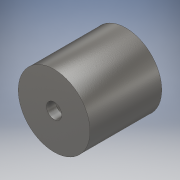
# Autodesk Inventor part: SensorHalter
Saved by Autodesk Inventor 2018.3 (Build 223284000, 284)
## iProperties
Created: 2020-01-09
Part Number: SensorHalter
Material: Generisch
Document SubType Name: Modeling
Designer: DerLobre
Density: 1 g/cm^3
Appearance: Galvanisiert
Author: DerLobre
Autodesk Inventor part; units mm, degrees
ref_plane "YZ Plane" through (0, 0, 0) normal (1, 0, 0) x (0, 1, 0)
ref_plane "XZ Plane" through (0, 0, 0) normal (0, 1, 0) x (-1, 0, 0)
ref_plane "XY Plane" through (0, 0, 0) normal (0, 0, 1) x (1, 0, 0)
sketch "Skizze1" plane through (0, 0, 0) normal (1, 0, 0) x (0, 1, 0)
  line L0 (-20, 8.1439) -> (-20, -11.8561)
  line L1 (-20, -11.8561) -> (20, -11.8561)
  line L2 (20, -11.8561) -> (20, -1.8561)
  line L3 (20, -1.8561) -> (-15, 2.1439)
  line L4 (-15, 2.1439) -> (-15, 8.1439)
  line L5 (-15, 8.1439) -> (-20, 8.1439)
  line L6 (0, -15.8561) -> (0, 12.1439) projected
  line L7 (-28, 0) -> (28, 0) projected
  point P0 (0, 0)
  dimension "d0" = 6
  dimension "d1" = 20
  dimension "d2" = 10
  dimension "d11" = 5
  dimension "d12" = 40
  constraints: 12 end point, 3 perpendicular, 1 parallel, 1 vertical, 1 other
  measures "d0" distance of L3.end L4.end
  measures "d1" distance of L0.start L0.end
  measures "d2" distance of L1.end L2.end
  measures "d11" distance of L4.end L0.start
  measures "d12" distance of L0.end L1.end
revolve "Umdrehung1" add sketch "Skizze1" angle 360 about axis through (0, -15, 8.1439) along (0, -1, 0)
sketch "Skizze2" plane through (0, -20, 8.1439) normal (0, -1, 0) x (1, 0, 0)
  point P0 (0, -8.1439)
  point P1 (0, 0)
hole "Bohrung1" at (0, -20, 8.1439) direction (0, 1, 0) diameter 8.5 end through all
